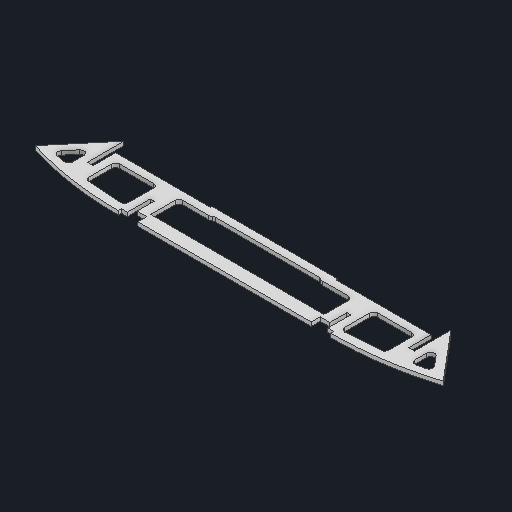
# Autodesk Inventor part: tail_2
Saved by Autodesk Inventor 2022.2 (Build 262287010, 287A)
## iProperties
Created: 2022-03-21
Part Number: tail_2
Material: Generic
Document SubType Name: Modeling
Designer: kardo
Density: 1 g/cm^3
Appearance: Default
Author: kardo
Autodesk Inventor part; units mm, degrees
ref_plane "YZ Plane" through (0, 0, 0) normal (1, 0, 0) x (0, 1, 0)
ref_plane "XZ Plane" through (0, 0, 0) normal (0, 1, 0) x (-1, 0, 0)
ref_plane "XY Plane" through (0, 0, 0) normal (0, 0, 1) x (1, 0, 0)
derived "parameters_frame.ipt"
derived "stencil_frame.ipt"
sketch "sk_joint_locations" plane through (81.12, 0, 0) normal (1, 0, 0) x (0, 1, 0)
  line L0 (0, 0) -> (135.09, 9.4464) construction
  line L1 (30.81, 28.832) -> (94.8, 28.832) construction
  arc A0 (30.81, 28.832) -> (9.48, 28.4869) centre (30.81, -630.4631) ccw construction
  line L2 (-254.1001, 19.9549) -> (9.48, 28.4869) construction
  line L3 (-363, 18.496) -> (-275.8801, 19.4795) construction
  arc A1 (-275.8801, 19.4795) -> (-254.1001, 19.9549) centre (-287.5515, 1053.3708) ccw construction
  line L4 (25.1322, 1581.9163) -> (267.6663, -1886.4825) construction
  line L5 (-242.0001, 1541.8302) -> (-242.0001, -1877.3857) construction
  line L6 (-120.9999, 1541.8302) -> (-120.9999, -1877.3857) construction
  line L7 (-363, 1541.8302) -> (-363, -1877.3857) construction
  line L8 (0, 1541.8302) -> (0, -1877.3857) construction
  line L9 (450.0665, 43.8884) -> (-613.9211, 6.7332) construction
  line L10 (-677.4829, -27.4989) -> (501.7293, 54.9597) construction
  line L11 (187.7215, 30.7247) -> (187.4423, 38.7198) construction
  line L12 (195.4031, 37.5588) -> (195.9625, 29.5588) construction
  line L13 (0, 3.808) -> (134.9306, 11.7256) construction
  line L14 (-242.0001, 45.8501) -> (-242.0001, 20.3465) construction
  line L15 (-363, 37.4293) -> (-363, 18.496) construction
  line L16 (-120.9999, 51.0063) -> (-120.9999, 24.2633) construction
  line L17 (0, 52.89) -> (0, 28.18) construction
  line L18 (132.2944, 49.425) -> (132.8217, 41.8851) construction
  line L19 (133.3489, 34.3453) -> (132.8217, 41.8851) construction
  line L20 (133.3489, 34.3453) -> (133.8761, 26.8054) construction
  line L21 (133.8761, 26.8054) -> (134.4034, 19.2655) construction
  line L22 (134.4034, 19.2655) -> (134.9306, 11.7256) construction
  line L23 (0, 3.808) -> (0, 0) construction
  spline S0 degree 4 poles (-363, 37.4293) (-272.3626, 45.1427) (-181.5879, 49.7528) (-90.8131, 52.89) (0, 52.89) knots 0 0 0 0 0 1 1 1 1 1
  spline S1 degree 3 poles (0, 52.89) (86.3106, 52.89) (181.3207, 49.5034) (237, 36.448) knots 0 0 0 0 1 1 1 1
  spline S2 degree 2 poles (135.09, 9.4464) (188.144, 13.1563) (237, 36.448) knots 0 0 0 1 1 1
  line L24 (94.8, 37.536) -> (94.8, 28.832) construction
  line L25 (94.8, 35.548) -> (94.8, 30.82) construction
  point P0 (187.5819, 34.7223)
  point P1 (195.6828, 33.5588)
  point P2 (134.9575, 11.3411)
  point P3 (-363, 27.9627)
  point P4 (-242.0001, 33.0983)
  point P5 (-120.9999, 37.6348)
  point P6 (0, 40.535)
  point P7 (94.8, 33.184)
sketch "sk_cowl_joint_locations" plane through (54.6, 0, 0) normal (1, 0, 0) x (0, 1, 0)
  line L0 (-363, 18.496) -> (-275.8801, 19.4795) construction
  arc A0 (-275.8801, 19.4795) -> (-254.1001, 19.9549) centre (-287.5515, 1053.3708) ccw construction
  line L1 (-254.1001, 19.9549) -> (9.48, 28.4869) construction
  arc A1 (30.81, 28.832) -> (9.48, 28.4869) centre (30.81, -630.4631) ccw construction
  line L2 (30.81, 28.832) -> (94.8, 28.832) construction
  line L3 (94.8, 30.032) -> (30.81, 30.032) construction
  arc A2 (30.81, 30.032) -> (9.4412, 29.6862) centre (30.81, -630.4631) ccw construction
  line L4 (9.4412, 29.6862) -> (-254.1389, 21.1542) construction
  arc A3 (-275.8936, 20.6794) -> (-254.1389, 21.1542) centre (-287.5515, 1053.3708) ccw construction
  line L5 (-275.8936, 20.6794) -> (-363, 19.6961) construction
  line L6 (-242.0001, 1541.8302) -> (-242.0001, -1877.3857) construction
  line L7 (-120.9999, 1541.8302) -> (-120.9999, -1877.3857) construction
  line L8 (-363, 1541.8302) -> (-363, -1877.3857) construction
  line L9 (0, 1541.8302) -> (0, -1877.3857) construction
  line L10 (-242.0001, 45.0688) -> (-242.0001, 21.5472) construction
  line L11 (-120.9999, 49.9661) -> (-120.9999, 25.4639) construction
  line L12 (-363, 19.6961) -> (-363, 19.6961)
  line L13 (-363, 19.6961) -> (-363, 36.9211) construction
  line L14 (-513.6167, 1550.4344) -> (344.3546, -1890.7004) construction
  line L15 (-362.7741, 36.9211) -> (-363, 39.712) construction
  line L16 (0, 51.6) -> (0, 29.3806) construction
  spline S0 degree 2 poles (-363, 39.712) (-181.6483, 54.394) (0, 54.4) knots 0 0 0 1 1 1
  spline S1 degree 3 poles (0, 54.4) (52.14, 54.4) (75.84, 49.3408) (94.8, 37.536) knots 1 1 1 1 2 2 2 2
  spline S2 degree 3 poles (93.3201, 35.1591) (91.7887, 36.1125) (88.6673, 37.9255) (84.5441, 39.9679) (80.1975, 41.8496) (76.5188, 43.2287) (71.6118, 44.7991) (67.4172, 45.9339) (61.7832, 47.203) (56.9422, 48.0997) (50.4217, 49.0741) (44.8094, 49.7373) (37.2484, 50.4231) (30.743, 50.8582) (21.9903, 51.263) (12.5916, 51.53) (4.3299, 51.6) (0, 51.6) knots 1 1 1 1 1.083333 1.166667 1.208333 1.291667 1.333333 1.416667 1.458333 1.541667 1.583333 1.666667 1.708333 1.791667 1.833333 1.916667 2 2 2 2
  spline S3 degree 3 poles (0, 51.6) (-20.1706, 51.5993) (-55.4643, 51.3605) (-95.7903, 50.6123) (-126.0307, 49.8474) (-146.1889, 49.2356) (-171.3841, 48.3435) (-191.5382, 47.528) (-216.7283, 46.3813) (-236.8783, 45.3621) (-262.0632, 43.9608) (-282.2091, 42.7379) (-307.3889, 41.082) (-332.5661, 39.2987) (-352.7052, 37.7363) (-362.7741, 36.9211) knots 0 0 0 0 0.166667 0.291667 0.333333 0.416667 0.458333 0.541667 0.583333 0.666666 0.708333 0.791666 0.833333 0.916666 1 1 1 1
  line L17 (-142.5135, 45.4866) -> (-137.389, 24.9334) construction
  line L18 (-134.789, 31.0394) -> (-138.6702, 30.0717) construction
  line L19 (-137.3512, 41.316) -> (-141.2324, 40.3483) construction
  line L20 (-142.5135, 45.4866) -> (-138.6324, 46.4543) construction
  line L21 (-137.389, 24.9334) -> (-133.5079, 25.9011) construction
  line L22 (-138.6324, 46.4543) -> (-138.8117, 52.2515) construction
  point P0 (0, 0)
  point P1 (-363, 28.3086)
  point P2 (-242.0001, 33.308)
  point P3 (-120.9999, 37.715)
  point P4 (0, 40.4903)
  point P5 (-513.6167, 1550.4344)
  point P6 (344.3546, -1890.7004)
  point P7 (-85.2629, 50.788)
  point P8 (0, 40.4903)
sketch "sk_tail_2_base" plane through (0, -242.0001, 0) normal (0, 1, 0) x (-1, 0, 0)
  spline S0 degree 2 poles (-54.6, 47.8729) (-109.262, 47.8729) (-156, 14.7183) knots 0 0 0 1 1 1 construction
  line L0 (0, 47.8729) -> (-54.6, 47.8729) construction
  line L1 (894.3992, -1153.6931) -> (-881.6022, 962.8628) construction
  line L2 (0, -1877.3857) -> (0, 1541.8302) construction
  line L3 (0, 20.7064) -> (-32.32, 20.7064)
  line L4 (-32.32, 20.7064) -> (-32.32, 21.5465)
  line L5 (-32.32, 21.5465) -> (-81.12, 21.5465)
  line L6 (-81.12, 21.5465) -> (-81.12, 33.0983)
  line L7 (-81.12, 33.0983) -> (-84.12, 33.0983)
  line L8 (-84.12, 33.0983) -> (-84.12, 14.3275)
  line L9 (-84.12, 14.3275) -> (-104.896, 39.0874)
  line L10 (0, 46.6729) -> (-54.6, 46.6729)
  line L11 (0, 46.6729) -> (0, 20.7064)
  spline S1 degree 5 poles (-54.6, 46.6729) (-65.235, 46.6727) (-75.8695, 45.884) (-86.4273, 44.246) (-107.4395, 39.1871) (-127.368, 30.8129) (-137.094, 25.7751) (-146.4079, 20.0514) (-155.3057, 13.7395) knots 0 0 0 0 0 0 0.493638 0.493638 0.493638 1 1 1 1 1 1
  point P0 (0, 0)
  point P1 (-34.32, 20.3465)
  point P2 (-34.32, 19.5064)
  dimension "d3" = 1.2
  dimension "d4" = 1.2
  dimension "d5" = 1.2
  dimension "d6" = 2
  dimension "d7" = 3
  dimension "d8" = 1.2
  constraints: 18 end point, 5 parallel, 4 perpendicular, 2 point on line, 1 coincident, 4 other
  measures "d4" distance from line of L3 point (-34.32, 19.506)
  measures "d5" distance from line of L5 point (-34.32, 20.347)
  measures "d6" distance from line of point (-34.32, 20.347) L4
  measures "d7" distance of L6.end L7.end
  measures "d8" distance between parallel lines of L1 L9
extrude "thicken" add sketch "sk_tail_2_base" along normal blind 2
sketch "sk_cut_joint" plane through (0, -242.0001, 0) normal (0, 1, 0) x (-1, 0, 0)
  line L0 (0, 47.8729) -> (-54.6, 47.8729) projected
  line L1 (-54.6, -1877.3857) -> (-54.6, 1541.8302) construction
  line L2 (-49.6, 47.8729) -> (-49.6, 33.308)
  line L3 (-49.6, 33.308) -> (-51.6, 33.308)
  line L4 (-51.6, 33.308) -> (-51.6, 47.8729)
  point P0 (0, 0)
  point P1 (-54.6, 33.308)
  dimension "d11" = 5
  dimension "d12" = 2
  constraints: 6 end point, 3 parallel, 3 point on line
  measures "d11" distance between parallel lines of L1 L2
  measures "d12" distance between parallel lines of L2 L4
extrude "cut_joint" cut sketch "sk_cut_joint" along normal through all both and the other way through all
sketch "sk_cut_liner" plane through (0, -242.0001, 0) normal (0, 1, 0) x (-1, 0, 0)
  line L0 (0, 47.8729) -> (-54.6, 47.8729) projected
  line L1 (-54.6, -1877.3857) -> (-54.6, 1541.8302) projected
  line L2 (-44.6, 47.8729) -> (-44.6, 42.0729)
  line L3 (-44.6, 42.0729) -> (-49.6, 42.0729)
  line L4 (-49.6, 42.0729) -> (-49.6, 45.0729)
  line L5 (-49.6, 45.0729) -> (-54.6, 45.0729)
  point P0 (0, 0)
  dimension "d13" = 3
  dimension "d14" = 2.8
  dimension "d15" = 5
  dimension "d17" = 5
  constraints: 8 end point, 4 parallel, 2 point on line
  measures "d13" distance between parallel lines of L3 L5
  measures "d14" distance between parallel lines of L0 L5
  measures "d15" distance between parallel lines of L1 L4
  measures "d17" distance between parallel lines of L2 L4
extrude "cut_liner" cut sketch "sk_cut_liner" along normal through all both and the other way through all
sketch "sk_cut_weight" plane through (0, -242.0001, 0) normal (0, 1, 0) x (-1, 0, 0)
  line L0 (-44.6, 47.8729) -> (-44.6, 42.0729) construction
  line L1 (-44.6, 42.0729) -> (-49.6, 42.0729) construction
  line L2 (-49.6, 42.0729) -> (-49.6, 45.0729) projected
  line L3 (-32.32, 21.5465) -> (-81.12, 21.5465) construction
  line L4 (-32.32, 20.7064) -> (-32.32, 21.5465) construction
  line L5 (0, 20.7064) -> (-32.32, 20.7064) construction
  line L6 (-81.12, 21.5465) -> (-81.12, 33.0983) construction
  line L7 (-84.12, 33.0983) -> (-84.12, 14.3275) construction
  spline S0 degree 3 poles (-54.6, 46.6729) (-57.6166, 46.6729) (-63.6125, 46.5204) (-71.0149, 45.9488) (-78.3481, 45.0915) (-84.1595, 44.1772) (-91.3552, 42.7486) (-97.057, 41.3771) (-104.1161, 39.3771) (-109.709, 37.5484) (-116.6326, 34.9765) (-122.1174, 32.6902) (-130.2638, 28.9171) (-140.9825, 23.2754) (-150.1426, 17.4021) (-155.3057, 13.7395) knots 0 0 0 0 0.083333 0.166667 0.208333 0.291667 0.333333 0.416667 0.458333 0.541667 0.583333 0.666667 0.708333 0.833333 1 1 1 1 construction
  line L8 (-84.12, 14.3275) -> (-104.896, 39.0874) construction
  line L9 (0, -1877.3857) -> (0, 1541.8302) projected
  line L10 (-88.12, 25.3174) -> (-88.12, 39.3855)
  line L11 (-88.12, 39.3855) -> (-98.1493, 37.2698)
  line L12 (-98.1493, 37.2698) -> (-88.12, 25.3174)
  line L13 (-88.12, 39.3855) -> (-88.12, 43.3855) construction
  line L14 (-98.1493, 37.2698) -> (-100.7205, 40.334) construction
  line L15 (0, 40.0729) -> (-44.6, 40.0729)
  line L16 (-44.6, 40.0729) -> (-44.6, 25.5465)
  line L17 (-44.6, 25.5465) -> (-28.32, 25.5465)
  line L18 (-28.32, 25.5465) -> (-28.32, 24.7064)
  line L19 (-28.32, 24.7064) -> (0, 24.7064)
  line L20 (-55.6, 42.6729) -> (-77.12, 41.185)
  line L21 (-77.12, 41.185) -> (-77.12, 25.5465)
  line L22 (-77.12, 25.5465) -> (-55.6, 25.5465)
  line L23 (-55.6, 25.5465) -> (-55.6, 42.6729)
  line L24 (-49.6, 42.0729) -> (-49.6, 21.5465) construction
  line L25 (-49.6, 42.0729) -> (-51.6, 42.0729) construction
  line L26 (-51.6, 42.0729) -> (-51.6, 21.5465) construction
  line L27 (-77.12, 41.185) -> (-77.3959, 45.1755) construction
  point P0 (0, 0)
  dimension "d22" = 2
  dimension "d23" = 4
  dimension "d24" = 4
  dimension "d25" = 4
  dimension "d26" = 4
  dimension "d28" = 4
  dimension "d29" = 4
  dimension "d30" = 4
  dimension "d31" = 4
  dimension "d32" = 4
  dimension "d33" = 4
  dimension "d34" = 4
  dimension "d35" = 2
  dimension "d39" = 4
  constraints: 36 end point, 11 parallel, 4 collinear, 4 point on line, 2 perpendicular, 3 other
  measures "d22" distance between parallel lines of L24 L26
  measures "d23" distance between parallel lines of L23 L26
  measures "d24" distance between parallel lines of L3 L22
  measures "d25" distance between parallel lines of L6 L21
  measures "d26" distance of L20.end L27.end
  measures "d28" distance between parallel lines of L7 L10
  measures "d29" distance between parallel lines of L8 L12
  measures "d30" distance of L10.end L13.end
  measures "d31" distance of L11.end L14.end
  measures "d32" distance between parallel lines of L5 L19
  measures "d33" distance between parallel lines of L4 L18
  measures "d34" distance between parallel lines of L3 L17
  measures "d35" distance between parallel lines of L1 L15
  measures "d39" vertical distance of L20.start point (-54.6, 46.673)
extrude "cut_weight" cut sketch "sk_cut_weight" along normal through all both and the other way through all
fillet "rounding" radius 2 10 edges at (28.32, -241.0001, 25.5465) (28.32, -241.0001, 24.7064) (44.6, -241.0001, 25.5465) (77.12, -241.0001, 41.185) (98.1493, -241.0001, 37.2698) (77.12, -241.0001, 25.5465) (88.12, -241.0001, 25.3174) (55.6, -241.0001, 25.5465) (55.6, -241.0001, 42.6729) (88.12, -241.0001, 39.3855)
mirror "mirror" about plane through (0, 0, 0) normal (1, 0, 0)
equation "\"d3\" = shell_thickness"
equation "\"d4\" = shell_thickness"
equation "\"d5\" = shell_thickness"
equation "\"d6\" = bulkhead_thickness"
equation "\"d7\" = stringer_thickness"
equation "\"d8\" = shell_thickness"
equation "\"d9\" = bulkhead_thickness"
equation "\"d11\" = cowl_liner_width"
equation "\"d12\" = bulkhead_thickness"
equation "\"d13\" = cowl_sealing_thickness"
equation "\"d14\" = cowl_shell_thickness + cowl_liner_thickness"
equation "\"d15\" = cowl_liner_width"
equation "\"d17\" = cowl_sealing_width"
equation "\"d22\" = bulkhead_thickness"
equation "\"d23\" = bulkhead_inset"
equation "\"d24\" = bulkhead_inset"
equation "\"d25\" = bulkhead_inset"
equation "\"d26\" = bulkhead_inset"
equation "\"d28\" = bulkhead_inset"
equation "\"d29\" = bulkhead_inset"
equation "\"d30\" = bulkhead_inset"
equation "\"d31\" = bulkhead_inset"
equation "\"d32\" = bulkhead_inset"
equation "\"d33\" = bulkhead_inset"
equation "\"d34\" = bulkhead_inset"
equation "\"d39\" = bulkhead_inset"
equation "\"d38\" = 0.5 * bulkhead_inset"
equation "\"shell_thickness\" = 1.2"
equation "\"stringer_thickness\" = 3"
equation "\"bulkhead_thickness\" = 2"
equation "\"cowl_liner_width\" = 5"
equation "\"cowl_sealing_thickness\" = 3"
equation "\"cowl_shell_thickness\" = 1.6"
equation "\"cowl_liner_thickness\" = 1.2"
equation "\"cowl_sealing_width\" = 5"
equation "\"bulkhead_inset\" = 4"
body "Solid1"
